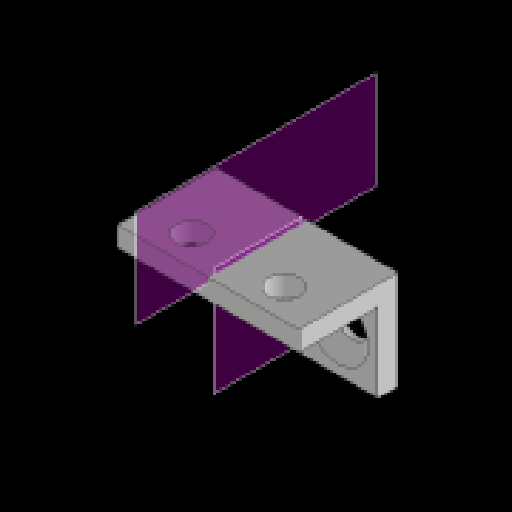
# Autodesk Inventor part: IRsensorHolder2
Saved by Autodesk Inventor 2024.3 (Build 283343010, 343A)
## iProperties
Created: 2025-04-16
Part Number: IRsensorHolder2
Material: Generic
Document SubType Name: Modeling
Designer: Oleg Kelner
Density: 1 g/cm^3
Appearance: Default
Author: Oleg Kelner
Autodesk Inventor part; units mm, degrees
ref_plane "YZ Plane" through (0, 0, 0) normal (1, 0, 0) x (0, 1, 0)
ref_plane "XZ Plane" through (0, 0, 0) normal (0, 1, 0) x (-1, 0, 0)
ref_plane "XY Plane" through (0, 0, 0) normal (0, 0, 1) x (1, 0, 0)
ref_plane "Work Plane1" through (-136.7474, 301.5, -3) normal (-1, 0, 0) x (0, 1, 0)
sketch "Sketch1" plane through (-136.7474, 301.5, -3) normal (-1, 0, 0) x (0, 1, 0)
  line L0 (-8.9333, -11.8308) -> (-8.9333, -1.8308)
  line L1 (-8.9333, -1.8308) -> (-18.9333, -1.8308)
  line L2 (-18.9333, -1.8308) -> (-18.9333, -3.8308)
  line L3 (-18.9333, -3.8308) -> (-10.9333, -3.8308)
  line L4 (-10.9333, -3.8308) -> (-10.9333, -11.8308)
  line L5 (-10.9333, -11.8308) -> (-8.9333, -11.8308)
  point P0 (-301.5, -3)
  point P1 (-8.9333, -6.8308)
  dimension "d0" = 10
  dimension "d1" = 10
  dimension "d2" = 2
  dimension "d3" = 2
  constraints: 12 end point, 3 perpendicular, 2 parallel, 1 horizontal, 1 midpoint
  measures "d0" distance of L0.start L0.end
  measures "d1" distance of L0.end L1.end
  measures "d2" distance of L1.end L2.end
  measures "d3" distance from line of point (-8.933, -6.831) L4
extrude "Extrusion1" add sketch "Sketch1" along normal mid plane 18.35
sketch "Sketch2" plane through (-145.9224, 290.5667, 8.8308) normal (0, -1, 0) x (1, 0, 0)
  circle A0 centre (4.5, 4.6692) radius 1.6 projected
  circle A1 centre (13.85, 4.6692) radius 1.6 projected
  circle A2 centre (4.5, -3) radius 1.6
  circle A3 centre (13.85, -3) radius 1.6
  line L0 (0, -8) -> (0, 0) projected
  line L1 (18.35, 0) -> (18.35, -8) projected
  line L2 (18.35, 0) -> (0, 0) projected
  point P0 (145.9224, -8.8308)
  dimension "d6" = 3.2
  dimension "d7" = 3.2
  dimension "d8" = 4.5
  dimension "d9" = 4.5
  dimension "d10" = 3
  dimension "d11" = 3
  constraints: 2 centre point
  measures "d6" diameter of A2
  measures "d7" diameter of A3
  measures "d8" distance from line of L0 A2.centre
  measures "d9" distance from line of L1 A3.centre
  measures "d10" distance from line of L2 A2.centre
  measures "d11" distance from line of L2 A3.centre
extrude "Extrusion2" cut sketch "Sketch2" against normal through all contours A2 | A3
sketch "Sketch3" plane through (-145.9224, 290.5667, 0.8308) normal (0, 0, 1) x (1, 0, 0)
  line L0 (18.35, -8) -> (0, -8) projected
  line L1 (18.35, 0) -> (18.35, -8) projected
  line L2 (0, -8) -> (0, 0) projected
  point P0 (145.9224, -290.5667)
  point P1 (4, -4)
  point P2 (14.35, -4)
  dimension "d14" = 4
  dimension "d15" = 4
  dimension "d16" = 4
  dimension "d17" = 4
  measures "d14" distance from line of L0 point (4, -4)
  measures "d15" distance from line of L0 point (14.35, -4)
  measures "d16" distance from line of L1 point (14.35, -4)
  measures "d17" distance from line of L2 point (4, -4)
hole "Hole1" at (-141.9224, 286.5667, 0.8308) at (-131.5724, 286.5667, 0.8308) direction (0, 0, -1) diameter 3.2 end through all countersink diameter 6 countersink angle 90
ref_plane "Work Plane2" through (-136.7474, 301.5, -3) normal (-1, 0, 0) x (0, 0, 1)
sketch "Sketch4" plane through (-136.7474, 301.5, -3) normal (-1, 0, 0) x (0, 0, 1)
  line L0 (3.8308, -10.9333) -> (11.8308, -10.9333) projected
  line L1 (1.8308, -18.9333) -> (3.8308, -18.9333) projected
  line L2 (11.8308, -10.9333) -> (3.8308, -18.9333)
  point P0 (3, -301.5)
  constraints: 2 end point
extrude "Rib1" add sketch "Sketch4" along normal mid plane 1 rib yes fills toward (7.8308, -10.9833) open curves L0 L2 L1
fillet "Fillet1" radius 1 4 edges at (-137.2474, 286.5667, 0.8308) (-137.2474, 290.5667, 4.8308) (-136.2474, 286.5667, 0.8308) (-136.2474, 290.5667, 4.8308)
body "Solid1"
